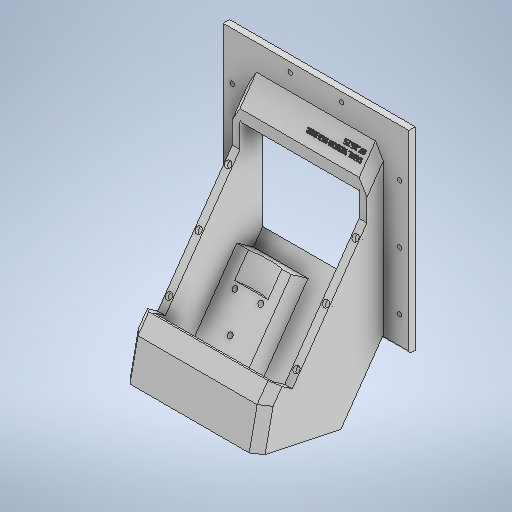
# Autodesk Inventor part: cameraholderbody v03
Saved by Autodesk Inventor 2025.2 (Build 292293000, 293)
## iProperties
Created: 2025-07-10
Part Number: cameraholderbody v03
Material: Generic
Document SubType Name: Modeling
Designer: mateo
Density: 1 g/cm^3
Appearance: Default
Author: mateo
Autodesk Inventor part; units mm, degrees
(part 1 of 2)
ref_plane "YZ Plane" through (0, 0, 0) normal (1, 0, 0) x (0, 1, 0)
ref_plane "XZ Plane" through (0, 0, 0) normal (0, 1, 0) x (-1, 0, 0)
ref_plane "XY Plane" through (0, 0, 0) normal (0, 0, 1) x (1, 0, 0)
sketch "Sketch1" plane through (0, 0, 0) normal (0, 0, 1) x (1, 0, 0)
  line L0 (40, -60) -> (-40, -60)
  line L1 (50, 50) -> (50, -50)
  line L2 (-50, -50) -> (-50, 50)
  line L3 (-40, 60) -> (40, 60)
  line L4 (50, -60) -> (50, 60)
  line L5 (50, 60) -> (-50, 60)
  line L6 (-50, 60) -> (-50, -60)
  line L7 (50, -60) -> (-50, -60)
  line L8 (-72, 82) -> (72, 82)
  line L9 (72, 82) -> (72, 0)
  line L10 (72, 0) -> (72, -82)
  line L11 (72, -82) -> (-72, -82)
  line L12 (-72, -82) -> (-72, 82)
  point P0 (0, 0)
  point P1 (0, 10)
  point P2 (0, 0)
  constraints: 26 end point, 3 perpendicular, 2 point on line, 1 collinear
extrude "Extrusion1" add sketch "Sketch1" along normal blind 5
sketch "Sketch2" plane through (0, 305, 5) normal (0, 0, 1) x (1, 0, 0)
  point P0 (0, 0)
  point P1 (-65, -305)
  point P2 (-65, -260)
  point P3 (-65, -350)
  point P4 (65, -305)
  point P5 (65, -260)
  point P6 (65, -350)
  point P7 (-20, -230)
  point P8 (20, -230)
  point P9 (-20, -380)
  point P10 (20, -380)
  dimension "d7" = 45
  dimension "d8" = 45
  dimension "d6" = 45
  dimension "d5" = 45
  measures "d7" distance of point (-65, -350) point (-65, -305)
  measures "d8" distance of point (-65, -305) point (-65, -260)
  measures "d6" distance of point (65, -305) point (65, -260)
  measures "d5" distance of point (65, -350) point (65, -305)
hole "Hole1" at (-65, 0, 5) at (-65, 45, 5) at (-65, -45, 5) at (65, 0, 5) at (65, 45, 5) at (65, -45, 5) at (-20, 75, 5) at (20, 75, 5) at (-20, -75, 5) at (20, -75, 5) direction (0, 0, -1) diameter 3.4587 depth 10.8 tip angle 118
move or copy body "Move Body1" bodies to move or copy 1 copy no translate (-2.5, -1.5, 0)
ref_plane "Work Plane1" through (-52.5, 58.5, 5) normal (0, -0.6427876, 0.7660444) x (1, 0, 0)
ref_plane "Work Plane2" through (47.5, -61.5, 5) normal (0, 0.5735764, 0.819152) x (-1, 0, 0)
sketch "Sketch6" plane through (47.5, -61.5, 5) normal (0, 0.5735764, 0.819152) x (-1, 0, 0)
  line L0 (102.232, 1.5875) -> (102.232, -110.9125)
  line L1 (-2.232, -110.9125) -> (-2.232, 1.5875)
  line L2 (-2.232, -110.9125) -> (102.232, -110.9125)
  line L3 (102.232, 1.5875) -> (102.232, 46.5875)
  line L4 (102.232, 46.5875) -> (-2.232, 46.5875)
  line L5 (-2.232, 46.5875) -> (-2.232, 1.5875)
  ellipse E0 centre (115, -12.2873) end of major axis (113.2706, -12.2873) minor radius 1.4166 projected
  ellipse E1 centre (-15, -12.2873) end of major axis (-16.7294, -12.2873) minor radius 1.4166 projected
  ellipse E2 centre (115, -49.1491) end of major axis (113.2706, -49.1491) minor radius 1.4166 projected
  ellipse E3 centre (-15, -49.1491) end of major axis (-16.7294, -49.1491) minor radius 1.4166 projected
  line L6 (102.232, 1.5875) -> (102.232, 46.5875)
  point P0 (47.5, -53.2457)
  dimension "d76" = 12.768
  dimension "d77" = 12.768
  dimension "d78" = 12.768
  dimension "d79" = 12.768
  constraints: 14 end point, 2 parallel, 2 perpendicular, 4 other
  measures "d76" distance from line of point (115, -12.287) L0
  measures "d77" distance from line of point (-15, -12.287) L1
  measures "d78" distance from line of L0 point (115, -49.149)
  measures "d79" distance from line of point (-15, -49.149) L1
extrude "Extrusion4" add sketch "Sketch6" along normal blind 70 contours L0 L2 L1 L5 L4 L3
sketch "Sketch8" plane through (47.5, -61.5, 5) normal (0, 0.5735764, 0.819152) x (-1, 0, 0)
  line L0 (0, -115.8875) -> (100, -115.8875) projected
  line L1 (0, -101.1661) -> (0, -2.8679) projected
  line L2 (96.232, -115.8875) -> (3.768, -115.8875)
  line L3 (102.232, 46.5875) -> (-2.232, 46.5875) projected
  line L4 (0, 46.5875) -> (100, 46.5875)
  line L5 (102.232, -110.9125) -> (102.232, -8.7172) projected
  line L6 (-2.232, -8.7172) -> (-2.232, -110.9125) projected
  line L7 (102.232, 0) -> (102.232, 46.5875) projected
  line L8 (96.232, 46.5875) -> (3.768, 46.5875)
  line L9 (3.768, 46.5875) -> (3.768, -115.8875)
  line L10 (3.768, -115.8875) -> (96.232, -115.8875)
  line L11 (96.232, -115.8875) -> (96.232, 46.5875)
  point P0 (47.5, -53.2457)
  point P1 (0, -8.7172)
  point P2 (96.232, -115.8875)
  point P3 (96.232, 46.5875)
  point P4 (3.768, 46.5875)
  point P5 (3.768, -115.8875)
  dimension "d42" = 6
  dimension "d43" = 6
  constraints: 12 end point, 2 horizontal, 2 parallel, 2 point on line, 1 perpendicular
  measures "d42" distance between parallel lines of L11 L5
  measures "d43" distance between parallel lines of L9 L6
extrude "Extrusion6" cut sketch "Sketch8" along normal blind 65
sketch "Sketch12" plane through (-54.732, -54.3593, 0) normal (-1, 0, 0) x (0, 0, 1)
  line L0 (0, 0) -> (0, 122.0413) projected
  line L1 (-1.2762, 123.8638) -> (0, 122.0413) projected
  line L2 (0, 122.0413) -> (-1.2762, 123.8638)
  line L3 (-1.2762, 123.8638) -> (-58.6698, 83.6763)
  line L4 (-58.6698, 83.6763) -> (0, -0.1129)
  line L5 (0, -0.1129) -> (0, 122.0413)
  point P0 (0, 54.3593)
  point P1 (0, 0)
  constraints: 8 end point, 2 perpendicular, 1 collinear, 1 vertical
extrude "Extrusion8" cut sketch "Sketch12" against normal through all
chamfer "Chamfer1" distance 6 angle 45 2 edges at (49.732, 0.5147, 47.0311) (-54.732, 0.5147, 47.0311)
sketch "Sketch15" plane through (47.5, -61.5, 5) normal (0, 0.5735764, 0.819152) x (-1, 0, 0)
  line L0 (96.232, -110.9125) -> (96.232, 46.5875) projected
  line L1 (3.768, -23.8125) -> (96.232, -23.8125)
  line L2 (96.232, -23.8125) -> (96.232, 11.2719)
  line L3 (3.768, 46.5875) -> (3.768, -110.9125) projected
  line L4 (3.768, 20.6375) -> (3.768, 46.5875)
  line L5 (3.768, 46.5875) -> (96.232, 46.5875)
  line L6 (96.232, 46.5875) -> (96.232, 11.2719)
  line L7 (102.232, 0) -> (102.232, 46.5875) projected
  line L8 (3.768, 46.5875) -> (3.768, -23.8125)
  point P0 (47.5, -53.2457)
  point P1 (96.6, -101.5469)
  point P2 (96.232, 46.5875)
  point P3 (2.1357, -101.5469)
  point P4 (3.768, -110.9125)
  point P5 (96.6, -100.9795)
  point P6 (2.1357, -100.9795)
  constraints: 12 end point, 1 parallel, 4 other
extrude "Extrusion11" add sketch "Sketch15" along normal blind 5 and the other way blind 3
ref_plane "Work Plane3" through (-54.732, -59.5119, 89.0621) normal (0, 0.819152, -0.5735764) x (1, 0, 0)
sketch "Sketch17" plane through (-54.732, -59.5119, 89.0621) normal (0, 0.819152, -0.5735764) x (1, 0, 0)
  line L0 (0, 70) -> (0, 6) projected
  line L1 (0, 6) -> (6, 0) projected
  line L2 (0, 6) -> (6, 0)
  line L3 (6, 0) -> (98.464, 0) projected
  line L4 (6, 0) -> (98.464, 0)
  line L5 (98.464, 0) -> (104.464, 6)
  line L6 (104.464, 6) -> (104.464, 34.8957)
  line L7 (104.464, 34.8957) -> (99.464, 34.8957)
  line L8 (6, 65) -> (6, 5) projected
  line L9 (0, 70) -> (0, 6) projected
  line L10 (0, 34.8957) -> (0, 6)
  line L11 (6, 5) -> (98.464, 5) projected
  line L12 (6, 5) -> (99.3003, 5)
  line L13 (98.464, 5) -> (98.464, 65) projected
  line L14 (6, 5) -> (6, 35)
  ellipse E0 centre (52.2321, 35) end of major axis (99.4643, 35) minor radius 30 (99.464, 34.8957) -> (99.464, 34.8957) ccw
  line L15 (99.464, 34.8957) -> (98.464, 34.8945)
  line L16 (98.464, 34.8945) -> (98.464, 5)
  line L17 (6, 5) -> (6, 35)
  line L18 (0, 34.8957) -> (6, 35)
  ellipse E1 centre (52.2319, 34.8945) end of major axis (5.9997, 34.8945) minor radius 30 (6, 35) -> (48.3586, 5) ccw
  ellipse E2 centre (52.2319, 34.8945) end of major axis (5.9997, 34.8945) minor radius 30 (56.1052, 5) -> (98.464, 34.8945) ccw
  point P0 (54.732, 38.8208)
  point P1 (5, 35)
  point P2 (5, 65)
  point P3 (0, 34.8957)
  point P4 (0, 34.8957)
  point P5 (6, 34.7891)
  point P6 (48.3586, 5)
  constraints: 24 end point, 4 perpendicular, 3 collinear, 3 point on line, 2 vertical, 16 other
extrude "Extrusion13" add sketch "Sketch17" against normal blind 15 contours L18 E0 L8 L11 L13 L7 L6 L5 L3 L1 L0 | L18 L8 E0 | L15 E0 L13 picked at (5.8412, 31.4681) picked at (98.6075, 31.369)
ref_plane "Work Plane4" through (-54.732, -99.6622, 31.7215) normal (0, -0.819152, 0.5735764) x (1, 0, 0)
ref_plane "Work Plane6" through (-54.732, -99.6622, 31.7215) normal (0, -0.9786416, 0.205574) x (1, 0, 0)
sketch "Sketch27" plane through (-54.732, -99.6622, 31.7215) normal (0, -0.9786416, 0.205574) x (1, 0, 0)
  line L0 (0, 38.1748) -> (5, 38.0788) projected
  line L1 (5, 38.0788) -> (0, 38.1748)
  line L2 (0, 4.6325) -> (0, 64.7463) projected
  line L3 (0, 38.1748) -> (0, 64.7463)
  line L4 (6, 70.2637) -> (0, 64.7463) projected
  line L5 (0, 64.7463) -> (6, 70.2637)
  line L6 (6, 70.2637) -> (98.425, 70.2637)
  line L7 (104.464, 64.7463) -> (104.464, 4.6325) projected
  line L8 (98.425, 70.2637) -> (104.464, 64.7463)
  line L9 (104.464, 64.7463) -> (104.464, 38.1748)
  line L10 (99.464, 38.1748) -> (104.464, 38.1748) projected
  line L11 (104.464, 38.1748) -> (99.464, 38.1748)
  line L12 (6, 1.5656) -> (6, 65.6659) projected
  ellipse E0 centre (52.2125, 38.1748) end of major axis (98.4632, 38.1748) minor radius 27.5938 (47.2131, 65.6069) -> (6, 39.2954) ccw
  line L13 (99.464, 38.1748) -> (99.4629, 38.3666)
  line L14 (99.4629, 38.3666) -> (99.464, 38.1748)
  line L15 (6, 65.6659) -> (98.464, 65.6659) projected
  line L16 (6, 65.6659) -> (57.4378, 65.5923)
  line L17 (99.3003, 65.6659) -> (6, 65.6659)
  line L18 (99.3003, 65.6659) -> (98.464, 65.6659)
  line L19 (98.464, 65.6659) -> (98.464, 38.1758) projected
  line L20 (99.464, 32.2809) -> (99.464, 38.1748) projected
  line L21 (5, 38.0788) -> (6, 38.0788) projected
  line L22 (5, 38.0788) -> (6, 38.0788)
  line L23 (6, 38.0788) -> (6, 65.6659)
  line L24 (98.464, 38.1758) -> (99.464, 38.1748) projected
  line L25 (98.464, 38.1758) -> (99.464, 38.1748)
  line L26 (99.464, 38.1748) -> (98.464, 38.1758)
  point P0 (54.732, -10.556)
  point P1 (48.3586, 65.6659)
  point P2 (56.1052, 65.6659)
  dimension "d91" = 5
  constraints: 32 end point, 7 collinear, 3 horizontal, 2 point on line, 1 perpendicular, 1 vertical, 7 other
  measures "d91" horizontal distance of L0.start L0.end
extrude "Extrusion21" add sketch "Sketch27" along normal mid plane 30 contours L2 L4 L6 L8 L7 L10 L24 L19 L15 L12 L21 L0
sketch "Sketch28" plane through (-54.732, -84.9826, 28.6379) normal (0, 0.9786416, -0.205574) x (1, 0, 0)
  line L0 (104.464, -64.7463) -> (104.464, -63.1884) projected
  line L1 (104.464, -64.7463) -> (104.464, -63.1884)
  line L2 (98.464, -6.7829) -> (98.464, -69.7132) projected
  line L3 (104.464, -63.1884) -> (98.464, -69.7132)
  line L4 (6, -6.7829) -> (6, -69.7132) projected
  line L5 (98.464, -69.7132) -> (6, -69.7132)
  line L6 (0, -63.1884) -> (6, -69.7132) projected
  line L7 (6, -69.7132) -> (0, -63.1884)
  line L8 (0, -63.1884) -> (0, -64.7463)
  line L9 (0, -64.7463) -> (6, -70.2637)
  line L10 (6, -70.2637) -> (98.464, -70.2637)
  line L11 (98.464, -70.2637) -> (104.464, -64.7463)
  point P0 (54.732, 10.556)
  constraints: 16 end point, 3 equal length, 3 perpendicular, 1 vertical
extrude "Extrusion22" cut sketch "Sketch28" against normal through all
sketch "Sketch31" plane through (-54.732, -61.5, 5) normal (-1, 0, 0) x (0, 0, 1)
  line L0 (26.7215, -38.1622) -> (55.4773, -18.0272) projected
  line L1 (64.0809, -30.3145) -> (67.1645, -44.9941) projected
  line L2 (26.7215, -38.1622) -> (67.1645, -44.9941)
  line L3 (55.4773, -18.0272) -> (64.0809, -30.3145) projected
  line L4 (67.0706, -45.0138) -> (94.0685, -39.3427) projected
  line L5 (70.081, -44.3815) -> (67.0706, -45.0138)
  line L6 (70.081, -44.3815) -> (63.7303, -15.5115)
  line L7 (63.7303, -15.5115) -> (25.4, -18.0272)
  line L8 (25.4, -18.0272) -> (26.7215, -38.1622)
  point P0 (-5, 61.5)
  point P1 (79.1472, -1.4534)
  constraints: 10 end point, 1 collinear, 1 perpendicular, 1 point on line
extrude "Extrusion25" add sketch "Sketch31" against normal blind 6
sketch "Sketch32" plane through (49.732, -61.5, 5) normal (1, 0, 0) x (0, 0, -1)
  line L0 (-26.7215, -38.1622) -> (0, 0) projected
  line L1 (-26.7215, -38.1622) -> (-67.1645, -44.9941) projected
  line L2 (-26.7215, -38.1622) -> (-67.1645, -44.9941)
  line L3 (-64.0809, -30.3145) -> (-67.1645, -44.9941) projected
  line L4 (-67.1645, -44.9941) -> (-64.0809, -30.3145)
  line L5 (-55.4773, -18.0272) -> (-64.0809, -30.3145) projected
  line L6 (-64.0809, -30.3145) -> (-55.4773, -18.0272)
  line L7 (-55.4773, -18.0272) -> (-26.7215, -38.1622)
  line L8 (-67.1645, -44.9941) -> (-71.4375, -44.0965)
  line L9 (-94.0685, -39.3427) -> (-67.1656, -44.9939) projected
  line L10 (-71.4375, -44.0965) -> (-64.617, -11.6275)
  line L11 (-64.617, -11.6275) -> (-26.7215, -38.1622)
  point P0 (5, 61.5)
  constraints: 14 end point, 3 collinear, 3 perpendicular, 2 point on line
extrude "Extrusion26" add sketch "Sketch32" against normal blind 6
sketch "Sketch34" plane through (47.5, -58.6321, 9.0958) normal (0, 0.5735764, 0.819152) x (1, 0, 0)
  line L0 (-3.768, 15.858) -> (-3.768, -46.5875) projected
  line L1 (-96.232, -46.5875) -> (-96.232, 15.858) projected
  line L2 (-96.232, -46.5875) -> (-3.768, -46.5875) projected
  line L3 (-3.768, 23.8125) -> (-96.232, 23.8125) projected
  line L4 (-50, -46.5875) -> (-50, 23.8125)
  line L5 (-94, -46.5875) -> (-54, -46.5875)
  line L6 (-54, -46.5875) -> (-54, 3.4125)
  line L7 (-54, 3.4125) -> (-94, 3.4125)
  line L8 (-94, 3.4125) -> (-96.232, 3.4125)
  line L9 (-96.232, 3.4125) -> (-96.232, -46.5875)
  line L10 (-94, -46.5875) -> (-96.232, -46.5875)
  point P0 (-47.5, 53.2457)
  point P1 (-54, -46.5875)
  dimension "d100" = 92.464
  dimension "d101" = 70.4
  dimension "d112" = 50
  constraints: 14 end point, 4 perpendicular, 2 midpoint, 2 point on line, 1 horizontal, 1 parallel
  measures "d100" distance between parallel lines of L0 L1
  measures "d101" distance between parallel lines of L2 L3
  measures "d112" distance between parallel lines of L2 L7
extrude "Extrusion27" add sketch "Sketch34" along normal blind 16
sketch "Sketch35" plane through (47.5, -49.4549, 22.2022) normal (0, 0.5735764, 0.819152) x (1, 0, 0)
  circle A0 centre (-74.6125, -42.8625) radius 2
  circle A1 centre (-84.6125, -19.1625) radius 2
  line L0 (-74.6125, 141.2434) -> (-74.6125, 78.7138)
  circle A2 centre (-64.6125, -19.1625) radius 2
  line L1 (-220.5298, -133.1321) -> (71.3048, -56.0245)
  point P0 (-47.5, 53.2457)
  point P1 (-90.1769, -210.863)
  point P2 (-74.6125, -94.5783)
  point P3 (-74.6125, -94.5783)
  dimension "d115" = 4
  dimension "d117" = 4
  dimension "d121" = 50
  dimension "d122" = 20
  dimension "d123" = 23.7
  constraints: 4 end point, 3 centre point, 2 midpoint, 2 vertical alignment, 1 symmetric about line, 1 vertical, 1 other
  measures "d115" diameter of A0
  measures "d117" diameter of A1
  measures "d121" distance from line of L1 A0.centre
  measures "d122" distance of A2.centre A1.centre
  measures "d123" vertical distance of A0.centre A1.centre
extrude "Extrusion28" cut sketch "Sketch35" against normal blind 24.6695
sketch "Sketch36" plane through (-74.5, -83.5, 5) normal (0, 0, 1) x (1, 0, 0)
  line L0 (22, 22) -> (19.768, 22) projected
  line L1 (124.232, 0) -> (19.768, 0)
  line L2 (124.232, 13.701) -> (19.768, 13.701)
  line L3 (19.768, 13.701) -> (0, 13.701)
  line L4 (0, 164) -> (0, 0) projected
  line L5 (0, 13.701) -> (0, 0)
  line L6 (0, 0) -> (19.768, 0)
  line L7 (0, 0) -> (144, 0) projected
  line L8 (124.232, 13.701) -> (144, 13.701)
  line L9 (144, 0) -> (144, 164) projected
  line L10 (144, 13.701) -> (144, 0)
  line L11 (144, 0) -> (124.232, 0)
  point P0 (74.5, 83.5)
  point P1 (0, 13.701)
  constraints: 16 end point, 3 collinear, 2 point on line, 1 perpendicular
sketch "Sketch37" plane through (-49.732, -99.6622, 31.7215) normal (0, -0.819152, 0.5735764) x (1, 0, 0)
  line L0 (-5, 0) -> (99.464, 0) projected
  line L1 (0, 8) -> (0, 0)
  line L2 (94.464, 0) -> (94.4704, 0)
  line L3 (-5, 0) -> (99.464, 0) projected
  line L4 (94.4704, 0) -> (94.464, 0)
  line L5 (93.464, 0) -> (93.464, 5)
  line L6 (93.464, 0) -> (93.464, 5) projected
  line L7 (93.464, 5) -> (43.232, 5)
  line L8 (43.232, 5) -> (43.232, 21)
  line L9 (43.232, 5) -> (93.464, 5) projected
  line L10 (0, 8) -> (0, 0)
  line L11 (1, 21) -> (4.232, 21)
  line L12 (1, 8) -> (1, 21)
  line L13 (1, 29.137) -> (1, 0) projected
  line L14 (1, -3) -> (1, 5) projected
  line L15 (0, 0) -> (0, -3)
  line L16 (93.464, -3) -> (93.464, 5) projected
  line L17 (1, -3) -> (93.464, -3)
  line L18 (93.464, -3) -> (93.464, 5)
  line L19 (1, 21) -> (43.232, 21)
  line L20 (-5, 0) -> (-5, 29.2104) projected
  line L21 (1, 21) -> (1, -3)
  line L22 (93.464, -3) -> (93.464, 5)
  line L23 (43.232, 5) -> (43.232, 21)
  point P0 (49.732, 31.1792)
  point P1 (0, 29.137)
  point P2 (1, 5)
  point P3 (0, 8)
  point P4 (93.464, 41.1414)
  point P5 (93.464, 65)
  point P6 (1, 29.2104)
  point P7 (93.464, 35.1055)
  point P8 (1, 0)
  point P9 (1, 0)
  point P10 (93.464, 0)
  constraints: 30 end point, 4 vertical, 3 collinear, 3 horizontal, 3 perpendicular, 1 point on line, 10 other
extrude "Extrusion29" add sketch "Sketch37" along normal blind 15
sketch "Sketch38" plane through (-49.732, -111.9495, 40.3251) normal (0, -0.819152, 0.5735764) x (1, 0, 0)
  line L0 (3.232, 8) -> (3.232, 24) projected
  line L1 (43.232, 5) -> (43.232, 21) projected
  line L2 (3.232, 24) -> (43.232, 24)
  line L3 (43.232, 24) -> (43.232, 22.05)
  line L4 (43.232, 22.05) -> (3.232, 22.05)
  line L5 (3.232, 22.05) -> (3.232, 24)
  point P0 (49.732, 31.1792)
  point P1 (3.232, 22.05)
  dimension "d141" = 16
  constraints: 8 end point, 2 parallel, 1 horizontal, 1 perpendicular, 1 point on line
  measures "d141" distance of L0.start L0.end
extrude "Extrusion30" cut sketch "Sketch38" against normal blind 288.2125
extrude "Extrusion31" cut sketch "Sketch36" against normal blind 288.2125
sketch "Sketch40" plane through (47.5, -61.5, 5) normal (0, -0.5735764, -0.819152) x (-1, 0, 0)
  circle A0 centre (74.6125, -42.8625) radius 2 projected
  circle A1 centre (64.6125, -19.1625) radius 2 projected
  circle A2 centre (84.6125, -19.1625) radius 2 projected
  circle A3 centre (74.6125, -42.8625) radius 5.5
  circle A4 centre (84.6125, -19.1625) radius 5.5
  circle A5 centre (64.6125, -19.1625) radius 5.5
  point P0 (47.5, 53.2457)
  dimension "d136" = 11
  dimension "d137" = 11
  dimension "d138" = 11
  constraints: 3 centre point, 3 coincident
  measures "d136" diameter of A3
  measures "d137" diameter of A4
  measures "d138" diameter of A5
extrude "Extrusion32" cut sketch "Sketch40" along normal blind 3
fillet "Fillet1" radius 2 1 edges at (-2.5, -69.799, 5)
sketch "Sketch41" plane through (47.5, -58.6321, 9.0958) normal (0, 0.5735764, 0.819152) x (1, 0, 0)
  line L0 (-54, 3.4125) -> (-54, -61.5875) projected
  line L1 (22, -5.1598) -> (-122, -5.1598) projected
  line L2 (-3.768, -61.5875) -> (-54, -61.5875) projected
  circle A0 centre (-29.5, -43.75) radius 3.5
  circle A1 centre (-29.5, -15.75) radius 3.5
  point P0 (-47.5, 53.2457)
  dimension "d147" = 7
  dimension "d149" = 7
  dimension "d196" = 28
  constraints: 2 centre point
  measures "d147" diameter of A0
  measures "d149" diameter of A1
  measures "d196" distance of A1.centre A0.centre
extrude "Extrusion33" cut sketch "Sketch41" against normal through all
sketch "Sketch42" plane through (47.5, -61.5, 5) normal (0, -0.5735764, -0.819152) x (-1, 0, 0)
  line L0 (97.232, -46.5875) -> (2.768, -46.5875) projected
  arc A0 (33, -43.75) -> (33, -43.75) centre (29.5, -43.75) ccw projected
  arc A1 (26, -43.75) -> (26, -43.75) centre (29.5, -43.75) ccw projected
  circle A2 centre (29.5, -43.75) radius 7.5
  circle A3 centre (29.5, -15.75) radius 3.5 projected
  circle A4 centre (29.5, -15.75) radius 7.5
  point P0 (47.5, 53.2457)
  point P1 (2.768, -46.5875)
  dimension "d158" = 15
  dimension "d197" = 15
  constraints: 2 centre point, 2 coincident, 1 other
  measures "d158" diameter of A2
  measures "d197" diameter of A4
extrude "Extrusion34" cut sketch "Sketch42" along normal blind 3
sketch "Sketch44" plane through (47.5, -61.5, 5) normal (0, -0.5735764, -0.819152) x (-1, 0, 0)
  line L0 (102.232, -46.5875) -> (96.232, -46.5875) projected
  line L1 (96.232, 0) -> (96.232, -46.5875) projected
  line L2 (102.232, 0) -> (102.232, -46.5875) projected
  line L3 (100, 0) -> (102.232, 0) projected
  line L4 (96.232, 0) -> (100, 0) projected
  line L5 (100, 8.7172) -> (96.232, 8.7172) projected
  line L6 (96.232, 8.7172) -> (96.232, 0) projected
  line L7 (100, 8.7172) -> (100, 0) projected
  line L8 (96.232, 0) -> (96.232, 2.1006) projected
  line L9 (102.232, -46.5875) -> (96.232, -46.5875)
  line L10 (96.232, -46.5875) -> (96.232, 0)
  line L11 (96.232, 0) -> (102.232, 0)
  line L12 (102.232, 0) -> (102.232, -46.5875)
  line L13 (3.768, -46.5875) -> (3.768, 0) projected
  line L14 (0, 0) -> (3.768, 0) projected
  line L15 (-2.232, 0) -> (0, 0) projected
  line L16 (-2.232, -46.5875) -> (-2.232, 0) projected
  line L17 (3.768, 8.7172) -> (0, 8.7172) projected
  line L18 (0, 0) -> (0, 8.7172) projected
  line L19 (3.768, 0) -> (3.768, 8.7172) projected
  line L20 (2.768, -46.5875) -> (-2.232, -46.5875)
  line L21 (-2.232, -46.5875) -> (-2.232, 0)
  line L22 (-2.232, 0) -> (2.768, 0)
  line L23 (2.768, 0) -> (2.768, -46.5875)
  line L24 (96.232, 0) -> (100, 0) projected
  line L25 (102.232, -46.5875) -> (96.232, -46.5875)
  line L26 (96.232, -46.5875) -> (96.232, 0)
  line L27 (96.232, 0) -> (102.232, 0)
  line L28 (102.232, 0) -> (102.232, -46.5875)
  line L29 (-2.232, -46.5875) -> (-2.232, 0) projected
  line L30 (2.768, -46.5875) -> (-2.232, -46.5875)
  line L31 (-2.232, -46.5875) -> (-2.232, 0)
  line L32 (-2.232, 0) -> (2.768, 0)
  line L33 (2.768, 0) -> (2.768, -46.5875)
  line L34 (96.232, 0) -> (96.232, -46.5875) projected
  line L35 (102.232, 0) -> (102.232, -46.5875) projected
  line L36 (100, 0) -> (102.232, 0) projected
  line L37 (96.232, 0) -> (100, 0) projected
  line L38 (3.768, -46.5875) -> (-2.232, -46.5875) projected
  line L39 (102.232, -46.5875) -> (96.232, -46.5875) projected
  line L40 (100, 8.7172) -> (96.232, 8.7172) projected
  line L41 (96.232, 8.7172) -> (96.232, 0) projected
  line L42 (100, 8.7172) -> (100, 0) projected
  line L43 (3.768, -46.5875) -> (3.768, 0) projected
  line L44 (0, 0) -> (3.768, 0) projected
  line L45 (-2.232, 0) -> (0, 0) projected
  line L46 (-2.232, -46.5875) -> (-2.232, 0) projected
  line L47 (3.768, -46.5875) -> (-2.232, -46.5875) projected
  line L48 (102.232, -46.5875) -> (96.232, -46.5875) projected
  line L49 (3.768, 8.7172) -> (0, 8.7172) projected
  line L50 (0, 0) -> (0, 8.7172) projected
  line L51 (3.768, 0) -> (3.768, 8.7172) projected
  point P0 (47.5, 53.2457)
  point P1 (102.232, -46.5875)
  point P2 (2.768, 0)
  constraints: 32 end point, 8 parallel, 4 horizontal, 4 perpendicular
extrude "Extrusion35" add sketch "Sketch44" along normal blind 3 contours L0 L1 L4 L3 L2 | L38 L23 L14 L13 | L20 L16 L15 L14 L23
sketch "Sketch45" plane through (44.732, -106.4941, 72.1645) normal (0, -0.9860303, -0.166566) x (1, 0, 0)
  line L0 (-99.464, -41.016) -> (-99.464, 0) projected
  line L1 (-99.464, -41.016) -> (5, -41.016) projected
  line L2 (5, 0) -> (5, -41.016) projected
  line L3 (-1, -33.9952) -> (-1, 0) projected
  line L4 (-1, -41.016) -> (5, -41.016) projected
  line L5 (-99.464, 0) -> (-93.464, 0)
  line L6 (-99.464, -41.016) -> (-99.464, 0)
  line L7 (5, 0) -> (5, -41.016) projected
  line L8 (0, 0) -> (5, 0)
  line L9 (5, 0) -> (5, -41.016)
  line L10 (-1, 0) -> (5, 0) projected
  line L11 (-1, -41.016) -> (-1, -33.9952) projected
  line L12 (5, -72.8496) -> (5, -43.1525) projected
  line L13 (5, -43.1525) -> (-99.464, -43.1525) projected
  line L14 (5, -43.1525) -> (-1, -43.1525)
  line L15 (-1, -43.1525) -> (-1, 0)
  line L16 (5, 0) -> (5, -43.1525)
  line L17 (5, -43.1525) -> (-99.464, -43.1525) projected
  line L18 (-99.464, -41.016) -> (-99.464, -43.1525)
  line L19 (-99.464, -43.1525) -> (-93.464, -43.1525)
  line L20 (-93.464, -43.1525) -> (-93.464, -41.016)
  line L21 (-93.464, 0) -> (-99.464, 0)
  line L22 (-99.464, 0) -> (-99.464, -43.1525)
  line L23 (-99.464, -43.1525) -> (-93.464, -43.1525)
  line L24 (-93.464, 0) -> (-93.464, -43.1525)
  line L25 (-93.464, -98.7163) -> (-93.464, 15.8051) projected
  point P0 (-44.732, -88.8947)
  point P1 (-94.464, -0.1031)
  point P2 (-94.464, -41.016)
  point P3 (-93.464, -0.1031)
  point P4 (5, -41.016)
  point P5 (-1, -41.016)
  point P6 (-93.464, -41.016)
  point P7 (-99.464, -41.016)
  constraints: 28 end point, 7 collinear, 3 horizontal, 1 perpendicular, 1 vertical
extrude "Extrusion37" add sketch "Sketch45" along normal blind 15 contours L0 L5 L24 L1 | L1 L20 L13 L18 | L11 L3 L10 L8 L2 L1 | L1 L16 L13 L15
sketch "Sketch47" plane through (49.732, -66.7303, 5) normal (1, 0, 0) x (0, 0, -1)
  line L0 (-67.0629, -39.7466) -> (-67.0706, -39.7835) projected
  line L1 (-67.0706, -39.7835) -> (-27.0245, -48.1956)
  line L2 (-64.6661, -54.5542) -> (-22.1163, -47.3665) projected
  line L3 (-27.0245, -48.1956) -> (-64.578, -54.5394)
  line L4 (-67.1645, -39.7638) -> (-94.0685, -34.1123) projected
  line L5 (-64.578, -54.5394) -> (-64.6661, -54.5542)
  line L6 (-67.1645, -39.7638) -> (-64.6661, -54.5542) projected
  line L7 (-67.1645, -39.7638) -> (-67.0706, -39.7835)
  point P0 (5, 66.7303)
  point P1 (-32.8677, -46.9399)
  point P2 (-24.223, -47.7224)
  point P3 (-63.9955, -25.144)
  constraints: 8 end point, 2 collinear, 1 point on line
extrude "Extrusion38" cut sketch "Sketch47" against normal blind 120
sketch "Sketch49" plane through (-48.732, -54.3593, 0) normal (-1, 0, 0) x (0, 0, 1)
  line L0 (0, 8.7172) -> (44.4209, -54.7224) projected
  line L1 (0, 8.7172) -> (0, -5.2303)
  line L2 (1.3377, -7.1407) -> (-11.1157, 10.6446) projected
  line L3 (-11.1157, 10.6446) -> (-4.3813, 15.3601)
  line L4 (-4.3813, 15.3601) -> (0, 8.7172)
  line L5 (0, 8.7172) -> (-4.5625, 15.2332) projected
  line L6 (-11.1157, 10.6446) -> (0, -5.2303)
  point P0 (0, 54.3593)
  constraints: 8 end point, 3 point on line, 2 perpendicular, 1 vertical
extrude "Extrusion40" cut sketch "Sketch49" against normal through all contours L1 L2 L3 L5
sketch "Sketch50" plane through (-48.732, -55.8368, 7.1384) normal (0, 0.819152, -0.5735764) x (1, 0, 0)
  line L0 (42.232, -16) -> (0, -16) projected
  line L1 (9.0575, -16) -> (7.9375, -16)
  arc A0 (34.925, -16) -> (9.0575, -16) centre (21.9913, -30.5193) ccw
  line L2 (34.925, -16) -> (9.0575, -16)
  point P0 (48.732, -26.1792)
  point P1 (33.6195, -16)
  point P2 (9.0575, -16)
  constraints: 4 end point, 2 point on circle, 2 point on line, 1 centre point
extrude "Extrusion41" cut sketch "Sketch50" against normal blind 18.575
sketch "Sketch52" plane through (-54.732, -66.7303, 5) normal (-1, 0, 0) x (0, 0, 1)
  line L0 (26.7215, -32.9319) -> (24.223, -47.7224) projected
  line L1 (27.0245, -48.1956) -> (94.0685, -34.1123) projected
  line L2 (24.223, -47.7224) -> (27.0245, -48.1956) projected
  line L3 (32.8677, -46.9399) -> (26.0097, -37.1457) projected
  line L4 (26.0097, -37.1457) -> (32.8677, -46.9399)
  line L5 (27.0245, -48.1956) -> (24.223, -47.7224)
  line L6 (26.0097, -37.1457) -> (24.223, -47.7224)
  line L7 (32.8677, -46.9399) -> (32.9391, -47.042)
  line L8 (32.9391, -47.042) -> (27.0245, -48.1956)
  point P0 (-5, 66.7303)
  point P1 (32.8849, -46.9646)
  constraints: 10 end point, 2 collinear, 1 perpendicular, 1 point on line
extrude "Extrusion43" cut sketch "Sketch52" against normal through all contours L3 L7 L1 L2 L0
sketch "Sketch53" plane through (-54.732, -66.7303, 5) normal (-1, 0, 0) x (0, 0, 1)
  line L0 (0, 116.8109) -> (85.4767, -5.2624) projected
  line L1 (12.7, 98.6735) -> (85.4767, -5.2624)
  line L2 (12.7, 81.631) -> (70.555, -0.9945)
  line L3 (12.7, 81.631) -> (12.7, 130.812)
  line L4 (70.555, -0.9945) -> (93.6625, 15.1855)
  line L5 (12.7, 130.812) -> (93.6625, 15.1855)
  line L6 (70.555, -0.9945) -> (12.7, 81.631)
  line L7 (12.7, 130.812) -> (12.7, 81.631)
  point P0 (-5, 66.7303)
  point P1 (87.7509, -8.5103)
  constraints: 14 end point, 2 collinear, 2 perpendicular, 2 point on line, 1 parallel
extrude "Extrusion44" cut sketch "Sketch53" against normal through all
sketch "Sketch56" plane through (-54.732, -66.7303, 5) normal (-1, 0, 0) x (0, 0, 1)
  line L0 (24.264, -34.6526) -> (22.1163, -47.3665) projected
  line L1 (24.223, -47.7224) -> (26.0097, -37.1457) projected
  line L2 (24.264, -34.6526) -> (26.0097, -37.1457)
  line L3 (26.0097, -37.1457) -> (24.223, -47.7224)
  line L4 (24.223, -47.7224) -> (21.9676, -47.3414)
  line L5 (21.9676, -47.3414) -> (24.264, -34.6526)
  point P0 (-5, 66.7303)
  constraints: 8 end point, 1 collinear, 1 perpendicular
extrude "Extrusion46" cut sketch "Sketch56" against normal through all contours L2 L1 L4 L0
sketch "Sketch57" plane through (43.732, -67.7248, 75.555) normal (0, 0.5735764, 0.819152) x (1, 0, 0)
  line L0 (6, 100.8671) -> (6, 0) projected
  line L1 (3.175, 90.4335) -> (3.175, 70.4335) construction
  line L2 (3.175, 70.4335) -> (3.175, 50.4335) construction
  line L3 (3.175, 50.4335) -> (3.175, 30.4335) construction
  line L4 (3.175, 30.4335) -> (3.175, 50.4335) construction
  line L5 (3.175, 30.4335) -> (3.175, 10.4335) construction
  line L6 (6, 0) -> (0, 0) construction
  line L7 (0, 100.8671) -> (6, 100.8671) construction
  circle A0 centre (3.175, 90.4335) radius 2.5
  circle A1 centre (3.175, 70.4335) radius 2.5
  circle A2 centre (3.175, 50.4335) radius 2.5
  circle A3 centre (3.175, 30.4335) radius 2.5
  circle A4 centre (3.175, 10.4335) radius 2.5
  line L8 (-98.464, 0) -> (-98.464, 100.8671) projected
  line L9 (6, 61.4258) -> (3.175, 61.4258)
  line L10 (0, 61.4258) -> (-92.464, 61.4258) projected
  line L11 (-50.232, 48.9803) -> (-50.232, -16.0197) projected
  circle A5 centre (-95.639, 90.4335) radius 2.5
  circle A6 centre (-95.639, 70.4335) radius 2.5
  circle A7 centre (-95.639, 50.4335) radius 2.5
  circle A8 centre (-95.639, 30.4335) radius 2.5
  circle A9 centre (-95.639, 10.4335) radius 2.5
  point P0 (3, 0)
  point P1 (3, 100.8671)
  dimension "d202" = 20
  dimension "d203" = 20
  dimension "d204" = 20
  dimension "d205" = 20
  dimension "d206" = 20
  dimension "d207" = 10.4335
  dimension "d208" = 10.4336
  dimension "d209" = 5
  dimension "d210" = 5
  dimension "d211" = 5
  dimension "d212" = 5
  dimension "d213" = 5
  constraints: 12 end point, 10 centre point, 5 coincident, 4 point on line, 2 midpoint, 2 vertical, 1 collinear
  measures "d202" distance of L1.start L1.end
  measures "d203" distance of L1.end L2.end
  measures "d204" distance of L2.end L3.end
  measures "d205" distance of L3.end L2.end
  measures "d206" distance of L3.end L5.end
  measures "d207" vertical distance of L5.end point (3, 0)
  measures "d208" vertical distance of L1.start point (3, 100.867)
  measures "d209" diameter of A0
  measures "d210" diameter of A1
  measures "d211" diameter of A2
  measures "d212" diameter of A3
  measures "d213" diameter of A4
sketch "Sketch58" plane through (47.5, -21.3496, 62.3406) normal (0, 0.5735764, 0.819152) x (1, 0, 0)
  line L0 (-6.4076, 82.6491) -> (-90.4873, 82.6491) construction
  line L1 (-90.4873, 82.6491) -> (-90.4873, 95.3086) construction
  line L2 (-90.4873, 95.3086) -> (-6.4076, 95.3086) construction
  line L3 (-6.4076, 95.3086) -> (-6.4076, 82.6491) construction
  spline S0 degree 2 poles (-9.1196, 86.4721) (-9.1196, 86.8895) (-8.7813, 87.5614) (-8.4972, 87.7491) knots 0 0 0 1 2 2 2
  spline S1 degree 2 poles (-8.4972, 87.7491) (-8.265, 87.8948) (-7.7883, 87.9936) (-7.4178, 87.9936) knots 0 0 0 1 2 2 2
  line L4 (-7.4178, 87.9936) -> (-6.7163, 87.9936)
  line L5 (-6.7163, 87.9936) -> (-6.7163, 84.9456)
  line L6 (-6.7163, 84.9456) -> (-7.4104, 84.9456)
  spline S2 degree 2 poles (-7.4104, 84.9456) (-7.8402, 84.9456) (-8.3292, 85.0741) (-8.5021, 85.1877) knots 0 0 0 1 2 2 2
  spline S3 degree 2 poles (-8.5021, 85.1877) (-8.7961, 85.3828) (-9.1196, 86.0275) (-9.1196, 86.4721) knots 0 0 0 1 2 2 2
  spline S4 degree 2 poles (-8.6973, 86.4672) (-8.6973, 86.1164) (-8.4651, 85.62) (-8.2354, 85.4792) knots 0 0 0 1 2 2 2
  spline S5 degree 2 poles (-8.2354, 85.4792) (-8.0724, 85.3828) (-7.7043, 85.2964) (-7.4302, 85.2964) knots 0 0 0 1 2 2 2
  line L7 (-7.4302, 85.2964) -> (-7.1214, 85.2964)
  line L8 (-7.1214, 85.2964) -> (-7.1214, 87.6429)
  line L9 (-7.1214, 87.6429) -> (-7.4302, 87.6429)
  spline S6 degree 2 poles (-7.4302, 87.6429) (-7.6994, 87.6429) (-8.1069, 87.5565) (-8.2724, 87.4404) knots 0 0 0 1 2 2 2
  spline S7 degree 2 poles (-8.2724, 87.4404) (-8.4848, 87.2971) (-8.6973, 86.8229) (-8.6973, 86.4672) knots 0 0 0 1 2 2 2
  spline S8 degree 2 poles (-10.6239, 88.0579) (-10.3547, 88.0579) (-9.9545, 87.9171) (-9.8137, 87.7763) knots 0 0 0 1 2 2 2
  spline S9 degree 2 poles (-9.8137, 87.7763) (-9.6532, 87.6182) (-9.5223, 87.1736) (-9.5223, 86.8476) knots 0 0 0 1 2 2 2
  line L10 (-9.5223, 86.8476) -> (-9.5223, 84.9456)
  line L11 (-9.5223, 84.9456) -> (-9.9273, 84.9456)
  line L12 (-9.9273, 84.9456) -> (-9.9273, 86.8476)
  spline S10 degree 2 poles (-9.9273, 86.8476) (-9.9273, 87.06) (-9.9817, 87.3465) (-10.0582, 87.4626) knots 0 0 0 1 2 2 2
  spline S11 degree 2 poles (-10.0582, 87.4626) (-10.1398, 87.5861) (-10.4213, 87.7121) (-10.6239, 87.7121) knots 0 0 0 1 2 2 2
  spline S12 degree 2 poles (-10.6239, 87.7121) (-10.8141, 87.7121) (-11.1105, 87.5861) (-11.192, 87.4626) knots 0 0 0 1 2 2 2
  spline S13 degree 2 poles (-11.192, 87.4626) (-11.2686, 87.3465) (-11.3229, 87.0624) (-11.3229, 86.8574) knots 0 0 0 1 2 2 2
  line L13 (-11.3229, 86.8574) -> (-11.3229, 84.9456)
  line L14 (-11.3229, 84.9456) -> (-11.728, 84.9456)
  line L15 (-11.728, 84.9456) -> (-11.728, 86.8476)
  spline S14 degree 2 poles (-11.728, 86.8476) (-11.728, 87.1662) (-11.5995, 87.6207) (-11.4365, 87.7763) knots 0 0 0 1 2 2 2
  spline S15 degree 2 poles (-11.4365, 87.7763) (-11.2908, 87.9195) (-10.9055, 88.0579) (-10.6239, 88.0579) knots 0 0 0 1 2 2 2
  line L16 (-11.9799, 87.9936) -> (-13.0074, 84.9456)
  line L17 (-13.0074, 84.9456) -> (-13.5064, 84.9456)
  line L18 (-13.5064, 84.9456) -> (-14.5339, 87.9936)
  line L19 (-14.5339, 87.9936) -> (-14.1066, 87.9936)
  line L20 (-14.1066, 87.9936) -> (-13.83, 87.1415)
  line L21 (-13.83, 87.1415) -> (-12.6666, 87.1415)
  line L22 (-12.6666, 87.1415) -> (-12.3899, 87.9936)
  line L23 (-12.3899, 87.9936) -> (-11.9799, 87.9936)
  line L24 (-13.7188, 86.7957) -> (-13.247, 85.3606)
  line L25 (-13.247, 85.3606) -> (-12.7777, 86.7957)
  line L26 (-12.7777, 86.7957) -> (-13.7188, 86.7957)
  line L27 (-16.589, 87.9936) -> (-14.8229, 87.9936)
  line L28 (-14.8229, 87.9936) -> (-14.8229, 84.9456)
  line L29 (-14.8229, 84.9456) -> (-15.228, 84.9456)
  line L30 (-15.228, 84.9456) -> (-15.228, 87.633)
  line L31 (-15.228, 87.633) -> (-16.589, 87.633)
  line L32 (-16.589, 87.633) -> (-16.589, 87.9936)
  line L33 (-20.4274, 84.9456) -> (-19.3776, 87.9936)
  line L34 (-19.3776, 87.9936) -> (-18.9404, 87.9936)
  line L35 (-18.9404, 87.9936) -> (-17.8907, 84.9456)
  line L36 (-17.8907, 84.9456) -> (-18.3254, 84.9456)
  line L37 (-18.3254, 84.9456) -> (-19.1701, 87.4774)
  line L38 (-19.1701, 87.4774) -> (-20.0149, 84.9456)
  line L39 (-20.0149, 84.9456) -> (-20.4274, 84.9456)
  line L40 (-21.7809, 87.9936) -> (-20.6003, 87.9936)
  line L41 (-20.6003, 87.9936) -> (-20.6003, 87.6824)
  line L42 (-20.6003, 87.6824) -> (-20.9881, 87.6824)
  line L43 (-20.9881, 87.6824) -> (-20.9881, 85.2569)
  line L44 (-20.9881, 85.2569) -> (-20.6003, 85.2569)
  line L45 (-20.6003, 85.2569) -> (-20.6003, 84.9456)
  line L46 (-20.6003, 84.9456) -> (-21.7809, 84.9456)
  line L47 (-21.7809, 84.9456) -> (-21.7809, 85.2569)
  line L48 (-21.7809, 85.2569) -> (-21.3932, 85.2569)
  line L49 (-21.3932, 85.2569) -> (-21.3932, 87.6824)
  line L50 (-21.3932, 87.6824) -> (-21.7809, 87.6824)
  line L51 (-21.7809, 87.6824) -> (-21.7809, 87.9936)
  spline S16 degree 2 poles (-23.132, 88.048) (-22.8011, 88.048) (-22.3367, 87.9097) (-22.1317, 87.8109) knots 0 0 0 1 2 2 2
  line L52 (-22.1317, 87.8109) -> (-22.1317, 87.302)
  line L53 (-22.1317, 87.302) -> (-22.1613, 87.302)
  spline S17 degree 2 poles (-22.1613, 87.302) (-22.3614, 87.4898) (-22.8678, 87.6972) (-23.1024, 87.6972) knots 0 0 0 1 2 2 2
  spline S18 degree 2 poles (-23.1024, 87.6972) (-23.4383, 87.6972) (-23.7817, 87.4181) (-23.7817, 87.1884) knots 0 0 0 1 2 2 2
  spline S19 degree 2 poles (-23.7817, 87.1884) (-23.7817, 87.0056) (-23.6013, 86.7784) (-23.4062, 86.7216) knots 0 0 0 1 2 2 2
  spline S20 degree 2 poles (-23.4062, 86.7216) (-23.2654, 86.6821) (-23.0308, 86.6277) (-22.8554, 86.5833) knots 0 0 0 1 2 2 2
  spline S21 degree 2 poles (-22.8554, 86.5833) (-22.6973, 86.5413) (-22.4478, 86.4153) (-22.3515, 86.314) knots 0 0 0 1 2 2 2
  spline S22 degree 2 poles (-22.3515, 86.314) (-22.2577, 86.2128) (-22.1539, 85.9411) (-22.1539, 85.7632) knots 0 0 0 1 2 2 2
  spline S23 degree 2 poles (-22.1539, 85.7632) (-22.1539, 85.3927) (-22.7319, 84.8913) (-23.179, 84.8913) knots 0 0 0 1 2 2 2
  spline S24 degree 2 poles (-23.179, 84.8913) (-23.4359, 84.8913) (-23.8903, 84.9926) (-24.0855, 85.0889) knots 0 0 0 1 2 2 2
  line L54 (-24.0855, 85.0889) -> (-24.0855, 85.573)
  line L55 (-24.0855, 85.573) -> (-24.0558, 85.573)
  spline S25 degree 2 poles (-24.0558, 85.573) (-23.9101, 85.4396) (-23.4556, 85.242) (-23.2061, 85.242) knots 0 0 0 1 2 2 2
  spline S26 degree 2 poles (-23.2061, 85.242) (-22.9246, 85.242) (-22.5763, 85.5063) (-22.5763, 85.7212) knots 0 0 0 1 2 2 2
  spline S27 degree 2 poles (-22.5763, 85.7212) (-22.5763, 85.9139) (-22.7813, 86.1436) (-22.974, 86.1955) knots 0 0 0 1 2 2 2
  spline S28 degree 2 poles (-22.974, 86.1955) (-23.1024, 86.2301) (-23.4754, 86.319) (-23.5989, 86.356) knots 0 0 0 1 2 2 2
  spline S29 degree 2 poles (-23.5989, 86.356) (-23.9126, 86.4524) (-24.204, 86.8401) (-24.204, 87.1242) knots 0 0 0 1 2 2 2
  spline S30 degree 2 poles (-24.204, 87.1242) (-24.204, 87.3045) (-24.0583, 87.6503) (-23.9274, 87.7713) knots 0 0 0 1 2 2 2
  spline S31 degree 2 poles (-23.9274, 87.7713) (-23.7817, 87.9047) (-23.4112, 88.048) (-23.132, 88.048) knots 0 0 0 1 2 2 2
  line L56 (-25.6786, 87.9936) -> (-24.498, 87.9936)
  line L57 (-24.498, 87.9936) -> (-24.498, 87.6824)
  line L58 (-24.498, 87.6824) -> (-24.8858, 87.6824)
  line L59 (-24.8858, 87.6824) -> (-24.8858, 85.2569)
  line L60 (-24.8858, 85.2569) -> (-24.498, 85.2569)
  line L61 (-24.498, 85.2569) -> (-24.498, 84.9456)
  line L62 (-24.498, 84.9456) -> (-25.6786, 84.9456)
  line L63 (-25.6786, 84.9456) -> (-25.6786, 85.2569)
  line L64 (-25.6786, 85.2569) -> (-25.2908, 85.2569)
  line L65 (-25.2908, 85.2569) -> (-25.2908, 87.6824)
  line L66 (-25.2908, 87.6824) -> (-25.6786, 87.6824)
  line L67 (-25.6786, 87.6824) -> (-25.6786, 87.9936)
  spline S32 degree 2 poles (-28.3364, 85.2939) (-28.5093, 85.4965) (-28.7019, 86.0893) (-28.7019, 86.4696) knots 0 0 0 1 2 2 2
  spline S33 degree 2 poles (-28.7019, 86.4696) (-28.7019, 86.8401) (-28.5142, 87.4404) (-28.3364, 87.6429) knots 0 0 0 1 2 2 2
  spline S34 degree 2 poles (-28.3364, 87.6429) (-28.1486, 87.8553) (-27.6522, 88.0579) (-27.3533, 88.0579) knots 0 0 0 1 2 2 2
  spline S35 degree 2 poles (-27.3533, 88.0579) (-27.0446, 88.0579) (-26.5505, 87.8479) (-26.3702, 87.6429) knots 0 0 0 1 2 2 2
  spline S36 degree 2 poles (-26.3702, 87.6429) (-26.1949, 87.4404) (-26.0071, 86.8451) (-26.0071, 86.4696) knots 0 0 0 1 2 2 2
  spline S37 degree 2 poles (-26.0071, 86.4696) (-26.0071, 86.0868) (-26.1973, 85.5039) (-26.3727, 85.2939) knots 0 0 0 1 2 2 2
  spline S38 degree 2 poles (-26.3727, 85.2939) (-26.5505, 85.0914) (-27.047, 84.8814) (-27.3533, 84.8814) knots 0 0 0 1 2 2 2
  spline S39 degree 2 poles (-27.3533, 84.8814) (-27.6645, 84.8814) (-28.1635, 85.0988) (-28.3364, 85.2939) knots 0 0 0 1 2 2 2
  spline S40 degree 2 poles (-28.2796, 86.4696) (-28.2796, 86.1683) (-28.1486, 85.7015) (-28.0301, 85.5483) knots 0 0 0 1 2 2 2
  spline S41 degree 2 poles (-28.0301, 85.5483) (-27.9091, 85.3902) (-27.5682, 85.2322) (-27.3558, 85.2322) knots 0 0 0 1 2 2 2
  spline S42 degree 2 poles (-27.3558, 85.2322) (-27.1359, 85.2322) (-26.805, 85.3853) (-26.679, 85.5483) knots 0 0 0 1 2 2 2
  spline S43 degree 2 poles (-26.679, 85.5483) (-26.558, 85.7039) (-26.4295, 86.1732) (-26.4295, 86.4696) knots 0 0 0 1 2 2 2
  spline S44 degree 2 poles (-26.4295, 86.4696) (-26.4295, 87.0699) (-26.9334, 87.7071) (-27.3558, 87.7071) knots 0 0 0 1 2 2 2
  spline S45 degree 2 poles (-27.3558, 87.7071) (-27.7781, 87.7071) (-28.2796, 87.0699) (-28.2796, 86.4696) knots 0 0 0 1 2 2 2
  line L68 (-31.3276, 87.9936) -> (-30.8731, 87.9936)
  line L69 (-30.8731, 87.9936) -> (-29.5244, 85.3655)
  line L70 (-29.5244, 85.3655) -> (-29.5244, 87.9936)
  line L71 (-29.5244, 87.9936) -> (-29.1465, 87.9936)
  line L72 (-29.1465, 87.9936) -> (-29.1465, 84.9456)
  line L73 (-29.1465, 84.9456) -> (-29.722, 84.9456)
  line L74 (-29.722, 84.9456) -> (-30.9496, 87.3589)
  line L75 (-30.9496, 87.3589) -> (-30.9496, 84.9456)
  line L76 (-30.9496, 84.9456) -> (-31.3276, 84.9456)
  line L77 (-31.3276, 84.9456) -> (-31.3276, 87.9936)
  line L78 (-35.4673, 87.9936) -> (-35.0622, 87.9936)
  line L79 (-35.0622, 87.9936) -> (-35.0622, 86.5018)
  line L80 (-35.0622, 86.5018) -> (-33.6593, 86.5018)
  line L81 (-33.6593, 86.5018) -> (-33.6593, 87.9936)
  line L82 (-33.6593, 87.9936) -> (-33.2542, 87.9936)
  line L83 (-33.2542, 87.9936) -> (-33.2542, 84.9456)
  line L84 (-33.2542, 84.9456) -> (-33.6593, 84.9456)
  line L85 (-33.6593, 84.9456) -> (-33.6593, 86.1411)
  line L86 (-33.6593, 86.1411) -> (-35.0622, 86.1411)
  line L87 (-35.0622, 86.1411) -> (-35.0622, 84.9456)
  line L88 (-35.0622, 84.9456) -> (-35.4673, 84.9456)
  line L89 (-35.4673, 84.9456) -> (-35.4673, 87.9936)
  spline S46 degree 2 poles (-38.2411, 85.2939) (-38.414, 85.4965) (-38.6067, 86.0893) (-38.6067, 86.4696) knots 0 0 0 1 2 2 2
  spline S47 degree 2 poles (-38.6067, 86.4696) (-38.6067, 86.8401) (-38.419, 87.4404) (-38.2411, 87.6429) knots 0 0 0 1 2 2 2
  spline S48 degree 2 poles (-38.2411, 87.6429) (-38.0534, 87.8553) (-37.5569, 88.0579) (-37.2581, 88.0579) knots 0 0 0 1 2 2 2
  spline S49 degree 2 poles (-37.2581, 88.0579) (-36.9493, 88.0579) (-36.4553, 87.8479) (-36.275, 87.6429) knots 0 0 0 1 2 2 2
  spline S50 degree 2 poles (-36.275, 87.6429) (-36.0996, 87.4404) (-35.9119, 86.8451) (-35.9119, 86.4696) knots 0 0 0 1 2 2 2
  spline S51 degree 2 poles (-35.9119, 86.4696) (-35.9119, 86.0868) (-36.1021, 85.5039) (-36.2775, 85.2939) knots 0 0 0 1 2 2 2
  spline S52 degree 2 poles (-36.2775, 85.2939) (-36.4553, 85.0914) (-36.9518, 84.8814) (-37.2581, 84.8814) knots 0 0 0 1 2 2 2
  spline S53 degree 2 poles (-37.2581, 84.8814) (-37.5693, 84.8814) (-38.0682, 85.0988) (-38.2411, 85.2939) knots 0 0 0 1 2 2 2
  spline S54 degree 2 poles (-38.1843, 86.4696) (-38.1843, 86.1683) (-38.0534, 85.7015) (-37.9349, 85.5483) knots 0 0 0 1 2 2 2
  spline S55 degree 2 poles (-37.9349, 85.5483) (-37.8138, 85.3902) (-37.473, 85.2322) (-37.2605, 85.2322) knots 0 0 0 1 2 2 2
  spline S56 degree 2 poles (-37.2605, 85.2322) (-37.0407, 85.2322) (-36.7097, 85.3853) (-36.5838, 85.5483) knots 0 0 0 1 2 2 2
  spline S57 degree 2 poles (-36.5838, 85.5483) (-36.4627, 85.7039) (-36.3343, 86.1732) (-36.3343, 86.4696) knots 0 0 0 1 2 2 2
  spline S58 degree 2 poles (-36.3343, 86.4696) (-36.3343, 87.0699) (-36.8382, 87.7071) (-37.2605, 87.7071) knots 0 0 0 1 2 2 2
  spline S59 degree 2 poles (-37.2605, 87.7071) (-37.6829, 87.7071) (-38.1843, 87.0699) (-38.1843, 86.4696) knots 0 0 0 1 2 2 2
  line L90 (-40.8174, 87.9936) -> (-39.0513, 87.9936)
  line L91 (-39.0513, 87.9936) -> (-39.0513, 84.9456)
  line L92 (-39.0513, 84.9456) -> (-39.4564, 84.9456)
  line L93 (-39.4564, 84.9456) -> (-39.4564, 87.633)
  line L94 (-39.4564, 87.633) -> (-40.8174, 87.633)
  line L95 (-40.8174, 87.633) -> (-40.8174, 87.9936)
  spline S60 degree 2 poles (-43.5393, 86.4721) (-43.5393, 86.8895) (-43.2009, 87.5614) (-42.9169, 87.7491) knots 0 0 0 1 2 2 2
  spline S61 degree 2 poles (-42.9169, 87.7491) (-42.6847, 87.8948) (-42.208, 87.9936) (-41.8375, 87.9936) knots 0 0 0 1 2 2 2
  line L96 (-41.8375, 87.9936) -> (-41.136, 87.9936)
  line L97 (-41.136, 87.9936) -> (-41.136, 84.9456)
  line L98 (-41.136, 84.9456) -> (-41.8301, 84.9456)
  spline S62 degree 2 poles (-41.8301, 84.9456) (-42.2599, 84.9456) (-42.7489, 85.0741) (-42.9218, 85.1877) knots 0 0 0 1 2 2 2
  spline S63 degree 2 poles (-42.9218, 85.1877) (-43.2157, 85.3828) (-43.5393, 86.0275) (-43.5393, 86.4721) knots 0 0 0 1 2 2 2
  spline S64 degree 2 poles (-43.1169, 86.4672) (-43.1169, 86.1164) (-42.8848, 85.62) (-42.6551, 85.4792) knots 0 0 0 1 2 2 2
  spline S65 degree 2 poles (-42.6551, 85.4792) (-42.492, 85.3828) (-42.124, 85.2964) (-41.8498, 85.2964) knots 0 0 0 1 2 2 2
  line L99 (-41.8498, 85.2964) -> (-41.5411, 85.2964)
  line L100 (-41.5411, 85.2964) -> (-41.5411, 87.6429)
  line L101 (-41.5411, 87.6429) -> (-41.8498, 87.6429)
  spline S66 degree 2 poles (-41.8498, 87.6429) (-42.1191, 87.6429) (-42.5266, 87.5565) (-42.6921, 87.4404) knots 0 0 0 1 2 2 2
  spline S67 degree 2 poles (-42.6921, 87.4404) (-42.9045, 87.2971) (-43.1169, 86.8229) (-43.1169, 86.4672) knots 0 0 0 1 2 2 2
  line L102 (-43.979, 87.9936) -> (-43.979, 84.9456)
  line L103 (-43.979, 84.9456) -> (-45.8858, 84.9456)
  line L104 (-45.8858, 84.9456) -> (-45.8858, 85.3063)
  line L105 (-45.8858, 85.3063) -> (-44.3841, 85.3063)
  line L106 (-44.3841, 85.3063) -> (-44.3841, 86.1411)
  line L107 (-44.3841, 86.1411) -> (-45.7846, 86.1411)
  line L108 (-45.7846, 86.1411) -> (-45.7846, 86.5018)
  line L109 (-45.7846, 86.5018) -> (-44.3841, 86.5018)
  line L110 (-44.3841, 86.5018) -> (-44.3841, 87.633)
  line L111 (-44.3841, 87.633) -> (-45.8858, 87.633)
  line L112 (-45.8858, 87.633) -> (-45.8858, 87.9936)
  line L113 (-45.8858, 87.9936) -> (-43.979, 87.9936)
  line L114 (-48.6893, 87.9936) -> (-48.1632, 87.9936)
  line L115 (-48.1632, 87.9936) -> (-47.1999, 86.7809)
  line L116 (-47.1999, 86.7809) -> (-46.7355, 86.7809)
  line L117 (-46.7355, 86.7809) -> (-46.7355, 87.9936)
  line L118 (-46.7355, 87.9936) -> (-46.3304, 87.9936)
  line L119 (-46.3304, 87.9936) -> (-46.3304, 84.9456)
  line L120 (-46.3304, 84.9456) -> (-47.1159, 84.9456)
  spline S68 degree 2 poles (-47.1159, 84.9456) (-47.3777, 84.9456) (-47.7309, 85.0025) (-47.8915, 85.1062) knots 0 0 0 1 2 2 2
  spline S69 degree 2 poles (-47.8915, 85.1062) (-48.052, 85.2099) (-48.2373, 85.5335) (-48.2373, 85.7731) knots 0 0 0 1 2 2 2
  spline S70 degree 2 poles (-48.2373, 85.7731) (-48.2373, 86.1066) (-47.8964, 86.5586) (-47.605, 86.6672) knots 0 0 0 1 2 2 2
  line L121 (-47.605, 86.6672) -> (-48.6893, 87.9936)
  spline S71 degree 2 poles (-47.8149, 85.8052) (-47.8149, 85.6718) (-47.7211, 85.4668) (-47.6223, 85.4001) knots 0 0 0 1 2 2 2
  spline S72 degree 2 poles (-47.6223, 85.4001) (-47.5358, 85.3433) (-47.3061, 85.2964) (-47.1381, 85.2964) knots 0 0 0 1 2 2 2
  line L122 (-47.1381, 85.2964) -> (-46.7355, 85.2964)
  line L123 (-46.7355, 85.2964) -> (-46.7355, 86.4425)
  line L124 (-46.7355, 86.4425) -> (-47.0912, 86.4425)
  spline S73 degree 2 poles (-47.0912, 86.4425) (-47.2666, 86.4425) (-47.5457, 86.3807) (-47.642, 86.2844) knots 0 0 0 1 2 2 2
  spline S74 degree 2 poles (-47.642, 86.2844) (-47.7309, 86.2004) (-47.8149, 85.9633) (-47.8149, 85.8052) knots 0 0 0 1 2 2 2
  spline S75 degree 2 poles (-8.5268, 91.4881) (-8.5268, 92.3081) (-8.0501, 93.0763) (-7.5537, 93.0763) knots 0 0 0 1 2 2 2
  spline S76 degree 2 poles (-7.5537, 93.0763) (-7.0498, 93.0763) (-6.578, 92.2933) (-6.578, 91.4906) knots 0 0 0 1 2 2 2
  spline S77 degree 2 poles (-6.578, 91.4906) (-6.578, 90.6656) (-7.0547, 89.9023) (-7.5537, 89.9023) knots 0 0 0 1 2 2 2
  spline S78 degree 2 poles (-7.5537, 89.9023) (-8.0551, 89.9023) (-8.5268, 90.6928) (-8.5268, 91.4881) knots 0 0 0 1 2 2 2
  spline S79 degree 2 poles (-8.0032, 92.4168) (-8.0625, 92.2662) (-8.1119, 91.8018) (-8.1119, 91.4881) knots 0 0 0 1 2 2 2
  spline S80 degree 2 poles (-8.1119, 91.4881) (-8.1119, 91.1744) (-8.0625, 90.7125) (-8.0007, 90.5569) knots 0 0 0 1 2 2 2
  spline S81 degree 2 poles (-8.0007, 90.5569) (-7.939, 90.4013) (-7.7241, 90.2407) (-7.5537, 90.2407) knots 0 0 0 1 2 2 2
  spline S82 degree 2 poles (-7.5537, 90.2407) (-7.3832, 90.2407) (-7.1634, 90.4013) (-7.0992, 90.5618) knots 0 0 0 1 2 2 2
  spline S83 degree 2 poles (-7.0992, 90.5618) (-7.0374, 90.7175) (-6.993, 91.1917) (-6.993, 91.4906) knots 0 0 0 1 2 2 2
  spline S84 degree 2 poles (-6.993, 91.4906) (-6.993, 91.8117) (-7.0325, 92.2415) (-7.0967, 92.4094) knots 0 0 0 1 2 2 2
  spline S85 degree 2 poles (-7.0967, 92.4094) (-7.156, 92.5675) (-7.3758, 92.7379) (-7.5537, 92.7379) knots 0 0 0 1 2 2 2
  spline S86 degree 2 poles (-7.5537, 92.7379) (-7.7216, 92.7379) (-7.9414, 92.5774) (-8.0032, 92.4168) knots 0 0 0 1 2 2 2
  line L125 (-10.8314, 90.4211) -> (-9.5124, 93.0121)
  line L126 (-9.5124, 93.0121) -> (-9.0777, 93.0121)
  line L127 (-9.0777, 93.0121) -> (-10.4707, 90.3222)
  line L128 (-10.4707, 90.3222) -> (-8.8973, 90.3222)
  line L129 (-8.8973, 90.3222) -> (-8.8973, 89.9641)
  line L130 (-8.8973, 89.9641) -> (-10.8314, 89.9641)
  line L131 (-10.8314, 89.9641) -> (-10.8314, 90.4211)
  line L132 (-11.8589, 93.0121) -> (-11.3698, 93.0121)
  line L133 (-11.3698, 93.0121) -> (-11.3698, 92.4292)
  line L134 (-11.3698, 92.4292) -> (-11.8589, 92.4292)
  line L135 (-11.8589, 92.4292) -> (-11.8589, 93.0121)
  line L136 (-14.2005, 93.0121) -> (-12.7135, 93.0121)
  line L137 (-12.7135, 93.0121) -> (-12.7135, 92.7009)
  line L138 (-12.7135, 92.7009) -> (-13.2668, 92.7009)
  line L139 (-13.2668, 92.7009) -> (-13.2668, 90.6582)
  line L140 (-13.2668, 90.6582) -> (-12.7135, 90.6582)
  line L141 (-12.7135, 90.6582) -> (-12.7135, 90.3791)
  spline S87 degree 2 poles (-12.7135, 90.3791) (-13.0272, 90.3791) (-13.3236, 90.2012) (-13.3434, 89.9542) knots 0 0 0 1 2 2 2
  line L142 (-13.3434, 89.9542) -> (-13.6595, 89.9542)
  line L143 (-13.6595, 89.9542) -> (-13.6595, 92.7009)
  line L144 (-13.6595, 92.7009) -> (-14.2005, 92.7009)
  line L145 (-14.2005, 92.7009) -> (-14.2005, 93.0121)
  spline S88 degree 2 poles (-16.6878, 92.0241) (-16.6878, 92.2587) (-16.5322, 92.6564) (-16.4013, 92.7898) knots 0 0 0 1 2 2 2
  spline S89 degree 2 poles (-16.4013, 92.7898) (-16.2654, 92.9306) (-15.9245, 93.0763) (-15.7195, 93.0763) knots 0 0 0 1 2 2 2
  spline S90 degree 2 poles (-15.7195, 93.0763) (-15.5145, 93.0763) (-15.1761, 92.938) (-15.0477, 92.7997) knots 0 0 0 1 2 2 2
  spline S91 degree 2 poles (-15.0477, 92.7997) (-14.8896, 92.6342) (-14.7118, 92.0784) (-14.7118, 91.6733) knots 0 0 0 1 2 2 2
  spline S92 degree 2 poles (-14.7118, 91.6733) (-14.7118, 91.2757) (-14.8748, 90.6359) (-15.0452, 90.3988) knots 0 0 0 1 2 2 2
  spline S93 degree 2 poles (-15.0452, 90.3988) (-15.2107, 90.1666) (-15.7343, 89.9073) (-16.0777, 89.9073) knots 0 0 0 1 2 2 2